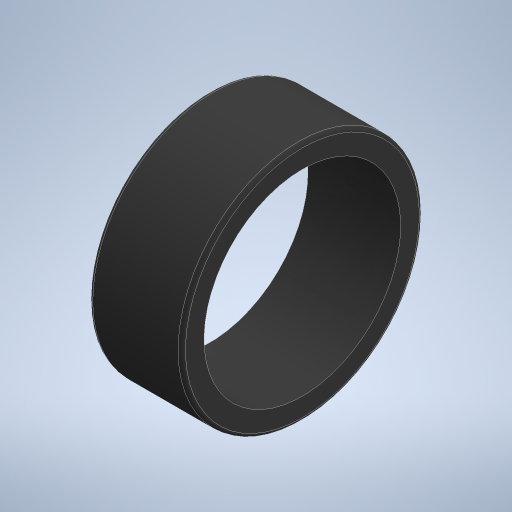
# Autodesk Inventor part: outertyre
Saved by Autodesk Inventor 2023 (Build 270158000, 158)
## iProperties
Created: 2022-11-29
Part Number: outertyre
Material: Rubber
Document SubType Name: Modeling
Designer: kakik
Density: 0.93 g/cm^3
Appearance: Rubber - Black
Author: kakik
Autodesk Inventor part; units mm, degrees
ref_plane "YZ Plane" through (0, 0, 0) normal (1, 0, 0) x (0, 1, 0)
ref_plane "XZ Plane" through (0, 0, 0) normal (0, 1, 0) x (-1, 0, 0)
ref_plane "XY Plane" through (0, 0, 0) normal (0, 0, 1) x (1, 0, 0)
sketch "Sketch1" plane through (0, 0, 0) normal (1, 0, 0) x (0, 1, 0)
  circle A0 centre (0, 0) radius 32.5
  circle A1 centre (0, 0) radius 26.5
  dimension "d0" = 65
  dimension "d1" = 6
  constraints: 2 centre point, 1 coincident
  measures "d0" diameter of A0
  measures "d1" radial gap between concentric circles of A0 A1
extrude "Extrusion1" add sketch "Sketch1" along normal blind 25
fillet "Fillet1" radius 1 2 edges at (0, -32.5, 0) (25, -32.5, 0)
body "Solid1"
